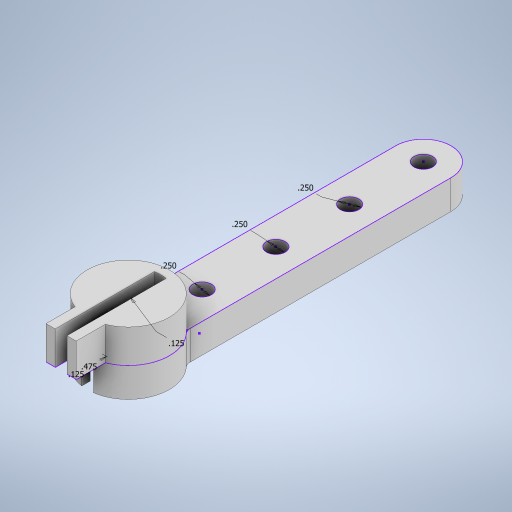
# Autodesk Inventor part: Torque Test Valve Lever
Saved by Autodesk Inventor 2023 (Build 270158000, 158)
## iProperties
Created: 2023-02-15
Part Number: Torque Test Valve Lever
Material: Generic
Document SubType Name: Modeling
Designer: tommy
Density: 1 g/cm^3
Appearance: Default
Author: tommy
Autodesk Inventor part; units mm, degrees
ref_plane "YZ Plane" through (0, 0, 0) normal (1, 0, 0) x (0, 1, 0)
ref_plane "XZ Plane" through (0, 0, 0) normal (0, 1, 0) x (-1, 0, 0)
ref_plane "XY Plane" through (0, 0, 0) normal (0, 0, 1) x (1, 0, 0)
sketch "Sketch1" plane through (0, 0, 0) normal (0, 1, 0) x (-1, 0, 0)
  arc A0 (-2.032, 11.0543) -> (2.032, 11.0543) centre (0, 0) ccw
  circle A1 centre (0, -25.4) radius 3.175
  circle A2 centre (0, -50.8) radius 3.175
  circle A3 centre (0, -76.2) radius 3.175
  circle A4 centre (0, -101.6) radius 3.175
  arc A5 (-9.525, -101.6) -> (9.525, -101.6) centre (0, -101.6) ccw
  line L0 (9.525, -101.6) -> (9.525, -11.7455)
  line L1 (-9.525, -11.7455) -> (-9.525, -101.6)
  arc A6 (10.369, -9.5897) -> (9.525, -11.7455) centre (12.7, -11.7455) ccw
  arc A7 (-9.525, -11.7455) -> (-10.369, -9.5897) centre (-12.7, -11.7455) ccw
  line L2 (-2.032, 11.0543) -> (-2.032, 13.9768)
  line L3 (2.032, 13.9768) -> (2.032, 11.0543)
  arc A8 (10.369, -9.5897) -> (2.032, 13.9768) centre (0, 0) ccw
  arc A9 (-2.032, 13.9768) -> (-10.369, -9.5897) centre (0, 0) ccw
  line L4 (-2.032, 11.0543) -> (-2.032, 23.1193)
  line L5 (-5.207, 23.1193) -> (-2.032, 23.1193)
  line L6 (-2.032, 23.1193) -> (-5.207, 23.1193)
  line L7 (-5.207, 23.1193) -> (-5.207, -13.1289)
  line L8 (-2.032, 23.1193) -> (-2.032, -13.9768)
  circle A10 centre (0, 0) radius 14.1237
  line L9 (0, 0) -> (0, -11.2395)
  line L10 (2.032, 11.0543) -> (2.032, 23.1193)
  line L11 (5.207, 23.1193) -> (2.032, 23.1193)
  line L12 (2.032, 23.1193) -> (5.207, 23.1193)
  line L13 (5.207, 23.1193) -> (5.207, -13.1289)
  line L14 (2.032, 23.1193) -> (2.032, -13.9768)
  point P0 (9.525, -10.4285)
  point P1 (-9.525, -10.4285)
  point P2 (-5.207, -9.9606)
  point P3 (-2.032, -11.0543)
  point P4 (5.207, -9.9606)
  point P5 (2.032, -11.0543)
  point P6 (5.207, 13.1289)
  point P7 (5.207, 9.9606)
  point P8 (-5.207, 9.9606)
  point P9 (-5.207, 13.1289)
  point P10 (2.032, 11.0543)
  point P11 (2.032, -11.0543)
  dimension "d9" = 6.35
  dimension "d10" = 6.35
  dimension "d11" = 6.35
  dimension "d12" = 3.175
  dimension "d15" = 12.065
  dimension "d16" = 3.175
  constraints: 30 end point, 20 point on circle, 11 centre point, 6 point on line, 4 symmetric about line, 3 tangent, 2 coincident, 1 equal radius, 1 parallel, 1 perpendicular, 1 vertical
  measures "d9" diameter of A1
  measures "d10" diameter of A2
  measures "d11" diameter of A3
  measures "d12" radius of A6
  measures "d15" distance of L2.start L4.end
  measures "d16" distance of L5.start L4.end
extrude "Extrusion1" add sketch "Sketch1" against normal blind 10.16 contours A0 L7 A9 L2 | A0 L7 A10 A9 | L8 A10 L7 A0 | A0 L14 A10 L8 | A8 L13 A0 L3 | A10 A6 L0 A5 L1 A7 | A8 A10 L13 A0 | A0 L13 A10 L14
extrude "Extrusion2" add sketch "Sketch1" along normal blind 11.43 contours L8 A0 L7 | A0 L7 A9 L2 | A9 L7 L5 L4 | L8 A10 L7 A0 | A8 L13 A0 L3 | L10 L11 L13 A8 | A0 L13 L14 | A0 L13 A10 L14
extrude "Extrusion3" add sketch "Sketch1" along normal blind 11.43 contours L7 A0 | A0 L7 A10 A9 | A0 L14 A10 L8 | A8 A10 L13 A0 | A0 L13
body "Solid1"
